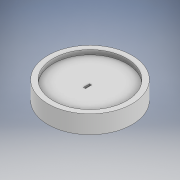
# Autodesk Inventor part: Knife_Centering_Jig_LM6013
Saved by Autodesk Inventor 2020.2 (Build 242310000, 310)
## iProperties
Created: 2020-04-05
Part Number: Knife_Centering_Jig_LM6013
Material: Generic
Document SubType Name: Modeling
Designer: rah75
Density: 1 g/cm^3
Appearance: Default
Author: rah75
Autodesk Inventor part; units mm, degrees
ref_plane "YZ Plane" through (0, 0, 0) normal (1, 0, 0) x (0, 1, 0)
ref_plane "XZ Plane" through (0, 0, 0) normal (0, 1, 0) x (-1, 0, 0)
ref_plane "XY Plane" through (0, 0, 0) normal (0, 0, 1) x (1, 0, 0)
sketch "Sketch1" plane through (0, 0, 0) normal (0, 1, 0) x (-1, 0, 0)
  circle A0 centre (0, 0) radius 12.065 construction
  circle A1 centre (0, 0) radius 12.215
  dimension "d0" = 24.13
  dimension "d1" = 0.15
  constraints: 2 centre point, 1 coincident
  measures "d0" diameter of A0
  measures "d1" radial gap between concentric circles of A0 A1
extrude "Extrusion1" add sketch "Sketch1" along normal mid plane 4.5
sketch "Sketch2" plane through (0, 0, 0) normal (1, 0, 0) x (0, 1, 0)
  line L0 (2.25, 1.7652) -> (-1.75, -0.1)
  line L1 (-1.75, -0.1) -> (2.25, -0.1)
  line L2 (2.25, -0.1) -> (2.25, 1.7652)
  line L3 (2.25, -12.215) -> (2.25, 12.215) projected
  line L4 (2.35, -0.2) -> (-2.2011, -0.2)
  line L5 (-2.2011, -0.2) -> (2.35, 1.9222)
  line L6 (2.35, 1.9222) -> (2.35, -0.2)
  point P0 (0, 0)
  dimension "d7" = 25
  dimension "d8" = 0.1
  dimension "d9" = 4
  dimension "d17" = 0.1
  constraints: 12 end point, 2 perpendicular, 1 collinear, 1 horizontal, 2 other
  measures "d7" angle of L1 L0
  measures "d8" distance from line of L1 point (0, 0)
  measures "d9" distance from line of L3 L0.end
  measures "d17" distance between parallel lines of L1 L4
extrude "Extrusion2" cut sketch "Sketch2" against normal mid plane 0.7
sketch "Sketch3" plane through (0, 2.25, 0) normal (0, 1, 0) x (1, 0, 0)
  circle A0 centre (0, 0) radius 12.215 projected
  circle A1 centre (0, 0) radius 13.965
  dimension "d12" = 1.75
  constraints: 1 centre point
  measures "d12" radial gap between concentric circles of A0 A1
extrude "Extrusion3" add sketch "Sketch3" along normal blind 1.5 and the other way blind 4.5
body "Solid1"
